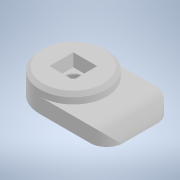
# Autodesk Inventor part: JBlock_plate
Saved by Autodesk Inventor 2021 (Build 250183000, 183)
## iProperties
Created: 2025-08-10
Part Number: JBlock_plate
Material: Generic
Catalog Web Link: www.cadenas.de
Description: JB LOCK PLATE-JB
Vendor: RITTAL
Document SubType Name: Modeling
Designer: psAdmin
Manufacturer: RITTAL
Mass: 2.84881 g
Surface Area: 16.896 cm^2
Volume: 2.84881 cm^3
Density: 1 g/cm^3
Appearance: PSOLRGB-175-175-175
Category: PARTsolutions
Company: RITTAL
Title: JBlock_plate
Author: Cadenas PARTsolutions
Comments: JB
PSOL_IDENT_0: {$CADENAS_DATA/23d-libs/rittal/schaltschranksys/kleingeh/jb_parts/lock_plate.prj},171 {VTYP=3D},{NB=
PSOL_IDENT_1: JBlock_plate},{LINA=JBlock_plate},{NN=JB LOCK PLATE},{DATE=20.08.2024 09:27:21},{GEOMDATE=03.07.2019
PSOL_IDENT_2: 13:23:23},{VERSION=},{LINEID=10},{WBVAR=},{WBNUMERIC=}  {NB=JBlock_plate},{LINA=JBlock_plate},{KT=D
PSOL_IDENT_3: UMMY},{PN=lock_plate},{DETAIL=MIN}
NB: JBlock_plate
NN: JB LOCK PLATE
NT: JB
NBSYN: JB$PN.
LINA: JBlock_plate
CATALOG: Rittal
PN: lock_plate
DETAIL: 0
SUPPLIER: RITTAL
ARTICLENO: JBlock_plate
BOMINFO: JBlock_plate
CREATOR: CADENAS GmbH
Autodesk Inventor part; units mm, degrees
sketch "Sketch_1" plane through (0, 0, 0) normal (0, 0, 1) x (1, 0, 0)
  line L0 (0, -10) -> (0, -2.65)
  line L1 (0, -2.65) -> (9, -2.65)
  line L2 (9, -2.65) -> (10, -3.65)
  line L3 (10, -3.65) -> (10, -10)
  line L4 (10, -10) -> (0, -10)
  line L5 (0, -10) -> (0, -2.65)
  constraints: 12 end point
revolve "Revolution1" add sketch "Sketch_1" angle 360 about axis through (0, -10, 0) along (0, -1, 0)
sketch "Sketch_2" plane through (0, -10, 0) normal (0, 1, 0) x (1, 0, 0)
  line L0 (0, 10) -> (0, -10)
  line L1 (0, -10) -> (15, -10)
  arc A0 (15, -10) -> (20, -5) centre (15, -5) ccw
  line L2 (20, -5) -> (20, 5)
  arc A1 (20, 5) -> (15, 10) centre (15, 5) ccw
  line L3 (15, 10) -> (0, 10)
  constraints: 8 end point, 4 point on circle, 2 centre point
extrude "Extrusion1" add sketch "Sketch_2" along normal blind 4.5
sketch "Sketch3" plane through (0, -10, -10) normal (0, -1, 0) x (1, 0, 0)
  point P0 (0, 10)
hole "Hole1" at (0, -10, 0) direction (0, 1, 0) diameter 5.5 depth 3.5 countersink diameter 11.7 countersink angle 90
sketch "Sketch_9" plane through (0, 0, 0) normal (0, 1, 0) x (-1, 0, 0)
  line L0 (3.55, -3.55) -> (3.55, 3.55)
  line L1 (3.55, 3.55) -> (-3.55, 3.55)
  line L2 (-3.55, 3.55) -> (-3.55, -3.55)
  line L3 (-3.55, -3.55) -> (3.55, -3.55)
  constraints: 8 end point
extrude "Extrusion2" cut sketch "Sketch_9" against normal blind 6.5
sketch "Sketch_3" plane through (0, 0, 0) normal (0, 0, 1) x (1, 0, 0)
  line L0 (15, -2) -> (15, -5.5)
  arc A0 (20, -10.5) -> (15, -5.5) centre (15, -10.5) ccw
  line L1 (20, -10.5) -> (25, -10.5)
  line L2 (25, -10.5) -> (25, -2)
  line L3 (25, -2) -> (15, -2)
  constraints: 8 end point, 2 point on circle, 1 centre point
extrude "Extrusion3" cut sketch "Sketch_3" along normal mid plane 20
ref_plane "bottom_to_ins_XY" through (0, 0, 0) normal (0, 1, 0) x (1, 0, 0)
ref_plane "bottom_to_ins_YZ" through (0, 0, 0) normal (1, 0, 0) x (0, 0, -1)
ref_plane "bottom_to_ins_ZX" through (0, 0, 0) normal (0, 0, -1) x (0, 1, 0)
body "Solid1"
